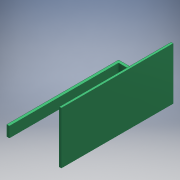
# Autodesk Inventor part: Porte Simple
Saved by Autodesk Inventor 2016 SP1 (Build 200210100, 210)
## iProperties
Created: 2016-10-04
Part Number: Porte Simple
Material: Bois (Chêne)
Document SubType Name: Modeling
Designer: dimercur
Density: 0.76 g/cm^3
Appearance: Lisse - Vert mer foncé
Mass: 1.7157e+06 g
Surface Area: 109150 cm^2
Volume: 2.2575e+06 cm^3
Author: dimercur
Autodesk Inventor part; units mm, degrees
ref_plane "YZ Plane" through (0, 0, 0) normal (1, 0, 0) x (0, 1, 0)
ref_plane "XZ Plane" through (0, 0, 0) normal (0, 1, 0) x (-1, 0, 0)
ref_plane "XY Plane" through (0, 0, 0) normal (0, 0, 1) x (1, 0, 0)
sketch "Esquisse1" plane through (0, 0, 0) normal (0, 0, 1) x (1, 0, 0)
  line L0 (-583.7545, 1063.2671) -> (466.2455, 1063.2671)
  line L1 (466.2455, 1063.2671) -> (466.2455, -1086.7329)
  line L2 (466.2455, -1086.7329) -> (-583.7545, -1086.7329)
  line L3 (-583.7545, -1086.7329) -> (-583.7545, 1063.2671)
  point P0 (0, 0)
  dimension "d0" = 1050
  dimension "d1" = 2150
  constraints: 8 end point, 2 parallel, 1 horizontal, 1 perpendicular
  measures "d0" distance of L0.start L0.end
  measures "d1" distance of L2.end L0.start
extrude "Extrusion1" add sketch "Esquisse1" along normal blind 1000
sketch "Esquisse2" plane through (-583.7545, 1063.2671, 0) normal (0, 1, 0) x (1, 0, 0)
  line L0 (0, 0) -> (0, -1000) projected
  line L1 (1050, -1000) -> (0, -1000) projected
  line L2 (0, -200) -> (1010, -200)
  line L3 (1010, -200) -> (1010, -1000)
  line L4 (1010, -1000) -> (0, -1000)
  line L5 (0, -1000) -> (0, -200)
  line L6 (1050, 0) -> (1050, -1000) projected
  point P0 (583.7545, 0)
  dimension "d4" = 200
  dimension "d5" = 40
  constraints: 8 end point, 2 parallel, 2 point on line, 1 horizontal, 1 perpendicular
  measures "d4" distance of L0.start L2.start
  measures "d5" distance between parallel lines of L6 L3
extrude "Extrusion2" cut sketch "Esquisse2" against normal through all
sketch "Esquisse3" plane through (-583.7545, 1063.2671, 200) normal (0, 0, 1) x (1, 0, 0)
  line L0 (1050, -2150) -> (0, -2150) projected
  line L1 (50, -50) -> (1010.0305, -50)
  line L2 (1010.0305, -50) -> (1010.0305, -2150)
  line L3 (1010.0305, -2150) -> (50, -2150)
  line L4 (50, -2150) -> (50, -50)
  line L5 (0, -2150) -> (0, 0) projected
  point P0 (583.7545, -1063.2671)
  dimension "d8" = 50
  dimension "d9" = 50
  constraints: 8 end point, 2 parallel, 1 horizontal, 1 perpendicular, 1 point on line
  measures "d8" distance between parallel lines of L5 L4
  measures "d9" horizontal distance of L1.start L5.end
extrude "Extrusion3" cut sketch "Esquisse3" against normal through all
